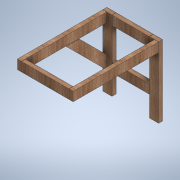
# Autodesk Inventor part: Frame Secondary
Saved by Autodesk Inventor 2020.2 (Build 242310000, 310)
## iProperties
Created: 2019-12-30
Part Number: Frame Secondary
Material: Wood (Birch)
Document SubType Name: Modeling
Designer: Andrew
Density: 0.1 g/cm^3
Appearance: Birch - Stained
Author: Andrew
Autodesk Inventor part; units mm, degrees
ref_plane "YZ Plane" through (0, 0, 0) normal (1, 0, 0) x (0, 1, 0)
ref_plane "XZ Plane" through (0, 0, 0) normal (0, 1, 0) x (-1, 0, 0)
ref_plane "XY Plane" through (0, 0, 0) normal (0, 0, 1) x (1, 0, 0)
derived "Desk Top Secondary.ipt"
sketch "Secondary Top" plane through (0, 0, 0) normal (0, 1, 0) x (-1, 0, 0)
  line L0 (0, 1270) -> (-143.3195, 1270)
  line L1 (-143.3195, 1270) -> (-143.3195, 0)
  line L2 (-143.3195, 0) -> (0, 0)
  line L3 (0, 0) -> (0, 1270)
  line L4 (-144.907, 1270) -> (-288.2265, 1270)
  line L5 (-288.2265, 1270) -> (-288.2265, 0)
  line L6 (-288.2265, 0) -> (-144.907, 0)
  line L7 (-144.907, 0) -> (-144.907, 1270)
  line L8 (-289.814, 1270) -> (-433.1335, 1270)
  line L9 (-433.1335, 1270) -> (-433.1335, 0)
  line L10 (-433.1335, 0) -> (-289.814, 0)
  line L11 (-289.814, 0) -> (-289.814, 1270)
  line L12 (-434.721, 1270) -> (-578.0405, 1270)
  line L13 (-578.0405, 1270) -> (-578.0405, 0)
  line L14 (-578.0405, 0) -> (-434.721, 0)
  line L15 (-434.721, 0) -> (-434.721, 1270)
sketch "Frame Secondary" plane through (0, 0, 0) normal (0, 1, 0) x (-1, 0, 0)
  line L0 (-53.9841, 898.525) -> (-524.0564, 898.525)
  line L1 (-524.0564, 898.525) -> (-524.0564, 858.8284)
  line L2 (-524.0564, 858.8284) -> (-53.9841, 858.8284)
  line L3 (-53.9841, 858.8284) -> (-53.9841, 898.525)
  line L4 (-12.7, 898.525) -> (-52.3966, 898.525)
  line L5 (-52.3966, 898.525) -> (-52.3966, 53.9841)
  line L6 (-52.3966, 53.9841) -> (-12.7, 53.9841)
  line L7 (-12.7, 53.9841) -> (-12.7, 898.525)
  line L8 (-12.7, 52.3966) -> (-103.759, 52.3966)
  line L9 (-103.759, 52.3966) -> (-103.759, 12.7)
  line L10 (-103.759, 12.7) -> (-12.7, 12.7)
  line L11 (-12.7, 12.7) -> (-12.7, 52.3966)
  line L12 (-105.3465, 52.3966) -> (-472.694, 52.3966)
  line L13 (-472.694, 52.3966) -> (-472.694, 12.7)
  line L14 (-472.694, 12.7) -> (-105.3465, 12.7)
  line L15 (-105.3465, 12.7) -> (-105.3465, 52.3966)
  line L16 (-565.3405, 12.7) -> (-474.2815, 12.7)
  line L17 (-474.2815, 12.7) -> (-474.2815, 52.3966)
  line L18 (-474.2815, 52.3966) -> (-565.3405, 52.3966)
  line L19 (-565.3405, 52.3966) -> (-565.3405, 12.7)
  line L20 (-565.3405, 53.9841) -> (-525.6439, 53.9841)
  line L21 (-525.6439, 53.9841) -> (-525.6439, 898.525)
  line L22 (-525.6439, 898.525) -> (-565.3405, 898.525)
  line L23 (-565.3405, 898.525) -> (-565.3405, 53.9841)
  point P0 (0, 0)
  point P1 (-578.0405, 1270)
  dimension "d1" = 39.6966
  dimension "d2" = 39.6966
  dimension "d3" = 39.6966
  dimension "d4" = 39.6966
  dimension "d5" = 91.059
  dimension "d6" = 91.059
  dimension "d7" = 1.5875
  dimension "d8" = 1.5875
  dimension "d9" = 1.5875
  dimension "d10" = 1.5875
  dimension "d11" = 1.5875
  dimension "d12" = 12.7
  dimension "d13" = 12.7
  dimension "d14" = 12.7
  dimension "d15" = 371.475
  constraints: 48 end point, 12 parallel, 8 point on line, 6 horizontal, 6 perpendicular, 1 collinear
  measures "d1" distance of L4.start L4.end
  measures "d2" distance of L10.end L8.start
  measures "d3" distance of L21.end L22.end
  measures "d4" distance of L2.end L0.start
  measures "d5" distance of L16.start L16.end
  measures "d6" distance of L9.end L10.end
  measures "d7" distance between parallel lines of L15 L9
  measures "d8" distance between parallel lines of L17 L13
  measures "d9" distance between parallel lines of L21 L1
  measures "d10" distance between parallel lines of L3 L5
  measures "d11" distance between parallel lines of L6 L8
  measures "d12" distance from line of point (0, 0) L7
  measures "d13" distance from line of point (-578.041, 1270) L23
  measures "d14" horizontal distance of L10.end point (0, 0)
  measures "d15" distance from line of point (-578.041, 1270) L0
extrude "Extrusion1" add sketch "Frame Secondary" against normal blind 91.059 contours L3 L2 L1 L0 | L7 L6 L5 L4 | L15 L14 L13 L12 | L23 L22 L21 L20
extrude "Extrusion2" add sketch "Frame Secondary" against normal blind 698.5 contours L11 L10 L9 L8 | L19 L18 L17 L16
derived "Desk Drawer.ipt"
derived "Frame Primary.ipt"
ref_plane "Support Plane" through (0, -495.3, 0) normal (0, 1, 0) x (-1, 0, 0)
extrude "Extrusion5" add sketch "Frame Secondary" along normal blind 91.059 from surface at -495.3 contours L15 L14 L13 L12
sketch "Sketch4" plane through (12.7, 0, 53.9841) normal (-1, 0, 0) x (0, 0, 1)
  line L0 (273.8766, -92.6465) -> (0, -366.5231)
  line L1 (0, -366.5231) -> (0, -495.3)
  line L2 (0, -495.3) -> (402.6535, -92.6465)
  line L3 (402.6535, -92.6465) -> (273.8766, -92.6465)
  line L4 (844.5409, -91.059) -> (0, -91.059) projected
  line L5 (-1.5875, 0) -> (-1.5875, -698.5) projected
  line L6 (-1.5875, -698.5) -> (-41.2841, -698.5) projected
  point P0 (-53.9841, 0)
  dimension "d24" = 1.5875
  dimension "d25" = 1.5875
  dimension "d26" = 45
  dimension "d27" = 203.2
  dimension "d28" = 91.059
  constraints: 8 end point, 1 parallel, 1 perpendicular
  measures "d24" distance between parallel lines of L3 L4
  measures "d25" distance between parallel lines of L5 L1
  measures "d26" angle of L5 L0
  measures "d27" distance from line of L6 L1.end
  measures "d28" distance between parallel lines of L2 L0
extrude "Angle Support" add sketch "Sketch4" against normal blind 39.6966 separate body
equation "\"d1\" = h_2x4"
equation "\"d2\" = h_2x4"
equation "\"d3\" = h_2x4"
equation "\"d4\" = h_2x4"
equation "\"d5\" = w_2x4"
equation "\"d6\" = w_2x4"
equation "\"d7\" = plank_tol"
equation "\"d8\" = plank_tol"
equation "\"d9\" = plank_tol"
equation "\"d10\" = plank_tol"
equation "\"d11\" = plank_tol"
equation "\"d13\" = d12"
equation "\"d14\" = d12"
equation "\"d16\" = w_2x4"
equation "\"d18\" = drawer_height"
equation "\"d33\" = w_2x4"
equation "\"d24\" = plank_tol"
equation "\"d25\" = plank_tol"
equation "\"d28\" = w_2x4"
equation "\"d29\" = h_2x4"
equation "\"h_2x4\" = 39.696571"
equation "\"w_2x4\" = 91.059"
equation "\"plank_tol\" = 1.5875"
equation "\"drawer_height\" = 698.5"
body "Solid1"
body "Solid2"
